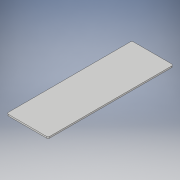
# Autodesk Inventor part: Maze Wall Cut Jig
Saved by Autodesk Inventor 2019 (Build 230136000, 136)
## iProperties
Created: 2019-02-13
Part Number: Maze Wall Cut Jig
Material: Generic
Document SubType Name: Modeling
Designer: Billy
Density: 1 g/cm^3
Appearance: Default
Author: Billy
Autodesk Inventor part; units mm, degrees
ref_plane "YZ Plane" through (0, 0, 0) normal (1, 0, 0) x (0, 1, 0)
ref_plane "XZ Plane" through (0, 0, 0) normal (0, 1, 0) x (-1, 0, 0)
ref_plane "XY Plane" through (0, 0, 0) normal (0, 0, 1) x (1, 0, 0)
sketch "Sketch1" plane through (0, 0, 0) normal (0, 1, 0) x (-1, 0, 0)
  line L0 (2, 0) -> (53, 0)
  line L1 (55, -2) -> (55, -164)
  line L2 (53, -166) -> (2, -166)
  line L3 (0, -164) -> (0, -2)
  arc A0 (53, -166) -> (55, -164) centre (53, -164) ccw
  arc A1 (0, -164) -> (2, -166) centre (2, -164) ccw
  arc A2 (55, -2) -> (53, 0) centre (53, -2) ccw
  arc A3 (2, 0) -> (0, -2) centre (2, -2) ccw
  point P0 (0, 0)
  point P1 (55, -166)
  point P2 (55, 0)
  point P3 (0, -166)
  dimension "d0" = 55
  dimension "d1" = 166
  dimension "d2" = 2
  constraints: 8 end point, 8 point on circle, 8 point on line, 8 tangent, 4 centre point, 3 equal radius, 2 parallel, 1 horizontal, 1 perpendicular
  measures "d0" distance of point (55, -166) point (0, -166)
  measures "d1" distance of point (55, 0) point (55, -166)
  measures "d2" radius of A0
extrude "Extrusion1" add sketch "Sketch1" along normal blind 2
body "Solid1"
